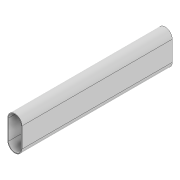
# Autodesk Inventor part: buis armsteun
Saved by Autodesk Inventor 2020.3 (Build 243373000, 373)
## iProperties
Created: 2020-09-11
Part Number: buis armsteun
Material: Generic
Document SubType Name: Modeling
Designer: Svend
Density: 1 g/cm^3
Appearance: Default
Author: Svend
Autodesk Inventor part; units mm, degrees
ref_plane "YZ Plane" through (0, 0, 0) normal (1, 0, 0) x (0, 1, 0)
ref_plane "XZ Plane" through (0, 0, 0) normal (0, 1, 0) x (-1, 0, 0)
ref_plane "XY Plane" through (0, 0, 0) normal (0, 0, 1) x (1, 0, 0)
sketch "Sketch1" plane through (0, 0, 0) normal (0, 0, 1) x (1, 0, 0)
  line L0 (-10, -14) -> (10, -14)
  line L1 (10, -14) -> (10, 14)
  line L2 (10, 14) -> (-10, 14)
  line L3 (-10, 14) -> (-10, -14)
  line L4 (-10, -14) -> (10, 14) construction
  line L5 (10, -14) -> (-10, 14) construction
  arc A0 (10, 14) -> (-10, 14) centre (0, 14) ccw
  arc A1 (-10, -14) -> (10, -14) centre (0, -14) ccw
  arc A2 (9, 14) -> (-9, 14) centre (0, 14) ccw
  arc A3 (-9, -14) -> (9, -14) centre (0, -14) ccw
  line L6 (-9, 14) -> (-9, -14)
  line L7 (9, 14) -> (9, -14)
  point P0 (0, 0)
  point P1 (0, -24)
  point P2 (0, 24)
  dimension "d0" = 20
  dimension "d1" = 48
  dimension "d2" = 1
  dimension "d3" = 1
  constraints: 16 end point, 12 point on circle, 4 centre point, 4 midpoint, 2 parallel, 2 vertical, 2 vertical alignment, 1 horizontal, 1 perpendicular
  measures "d0" distance of L1.end L2.end
  measures "d1" distance of point (0, 24) point (0, -24)
  measures "d2" radial gap between concentric circles of A0 A2
  measures "d3" radial gap between concentric circles of A1 A3
extrude "Extrusion1" add sketch "Sketch1" along normal mid plane 210 contours L3 L2 L6 L0 | L0 A3 A1 | A0 L2 A2 | L0 L7 L2 L1
body "Solid1"
